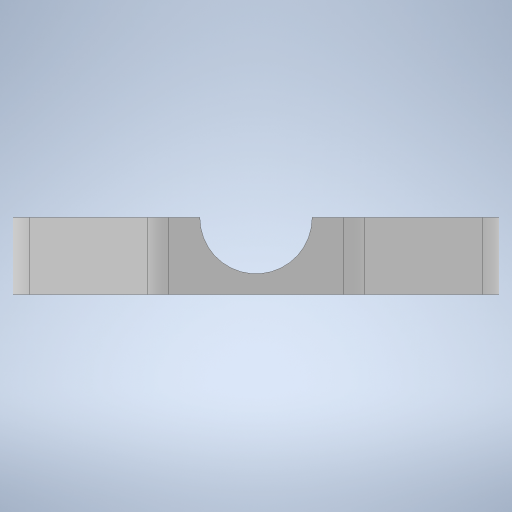
# Autodesk Inventor part: PlateSpacer6Hole - EndArmClamp
Saved by Autodesk Inventor 2023 (Build 270158000, 158)
## iProperties
Created: 2023-01-27
Part Number: PlateSpacer6Hole - EndArmClamp
Material: Generic
Document SubType Name: Modeling
Designer: chase
Density: 1 g/cm^3
Appearance: Default
Author: chase
Autodesk Inventor part; units mm, degrees
ref_plane "YZ Plane" through (0, 0, 0) normal (1, 0, 0) x (0, 1, 0)
ref_plane "XZ Plane" through (0, 0, 0) normal (0, 1, 0) x (-1, 0, 0)
ref_plane "XY Plane" through (0, 0, 0) normal (0, 0, 1) x (1, 0, 0)
sketch "Sketch1" plane through (0, 0, 0) normal (0, 0, 1) x (1, 0, 0)
  circle A0 centre (-11.2, 42.0257) radius 1.55
  circle A1 centre (0, 58.8568) radius 1.55
  circle A2 centre (-11.2, 16.8311) radius 1.55
  circle A3 centre (0, 8.9) radius 1.55
  circle A4 centre (0, 0) radius 1.55
  line L0 (-16.6, 4.9998) -> (-16.6, 54.9998) construction
  circle A5 centre (0, 50.2) radius 1.55
  line L1 (-11.2, 42.0257) -> (-11.2, 16.8311) construction
  line L2 (-16.6, 42.0257) -> (-16.6, 16.8311)
  line L3 (-5.8, 16.8311) -> (-5.8, 42.0257)
  arc A6 (-5.8, 42.0257) -> (-16.6, 42.0257) centre (-11.2, 42.0257) ccw
  arc A7 (-16.6, 16.8311) -> (-5.8, 16.8311) centre (-11.2, 16.8311) ccw
  line L4 (0, 58.8568) -> (0, 0) construction
  line L5 (-5.4, 58.8568) -> (-5.4, 0)
  line L6 (5.4, 0) -> (5.4, 58.8568)
  arc A8 (5.4, 58.8568) -> (-5.4, 58.8568) centre (0, 58.8568) ccw
  arc A9 (-5.4, 0) -> (5.4, 0) centre (0, 0) ccw
  line L7 (-15.6956, 45.0172) -> (-4.4956, 61.8483)
  line L8 (-15.6956, 13.8395) -> (-4.4956, -2.9916)
  point P0 (17, 90.5)
  point P1 (-11.2, 29.4284)
  point P2 (0, 29.4284)
  point P3 (-5.8, 29.2936)
  point P4 (-5.8, 29.2936)
  point P5 (-16.6, 29.4284)
  dimension "d2" = 0
  dimension "d3" = 0
  dimension "d4" = 0
  dimension "d5" = 0
  dimension "d6" = 16.6
  dimension "d7" = 5.4
  dimension "d8" = 5.4
  dimension "d9" = 5.4
  dimension "d10" = 3.1
  dimension "d11" = 3.1
  dimension "d12" = 3.1
  dimension "d13" = 3.1
  dimension "d14" = 3.1
  dimension "d15" = 3.1
  constraints: 22 end point, 12 point on circle, 12 tangent, 10 centre point, 3 midpoint, 3 vertical, 1 parallel, 1 point on line
  measures "d2" horizontal distance of A5.centre L4.start
  measures "d3" horizontal distance of A3.centre L4.start
  measures "d4" distance of point (0, 0) L4.end
  measures "d5" vertical distance of point (0, 29.428) point (-11.2, 29.428)
  measures "d6" distance from line of point (0, 0) L0
  measures "d7" radius of A6
  measures "d8" radius of A8
  measures "d9" radius of A9
  measures "d10" diameter of A2
  measures "d11" diameter of A0
  measures "d12" diameter of A5
  measures "d13" diameter of A1
  measures "d14" diameter of A4
  measures "d15" diameter of A3
extrude "Extrusion1" add sketch "Sketch1" along normal blind 11
sketch "Sketch2" plane through (-16.6, 16.8311, 0) normal (-1, 0, 0) x (0, 0, 1)
  line L0 (11, 25.1946) -> (11, 0) projected
  circle A0 centre (11, 12.5973) radius 8.05
  point P0 (0, -16.8311)
  dimension "d18" = 16.1
  constraints: 1 centre point, 1 midpoint
  measures "d18" diameter of A0
extrude "Extrusion2" cut sketch "Sketch2" against normal through all
equation "\"d8\" = d7"
equation "\"d9\" = d8"
equation "\"d11\" = d10"
equation "\"d12\" = d10"
equation "\"d13\" = d10"
equation "\"d14\" = d10"
equation "\"d15\" = d10"
body "Solid1"
